Autodesk Fusion 360 part; units mm, degrees
(part 2 of 2)
sketch "Sketch2" plane through (0, 0, 11) normal (0, 0, 1) x (1, 0, 0)
  circle A0 centre (16.996833, -24.059516) radius 1
  circle A1 centre (24.059516, -16.996833) radius 1
  circle A2 centre (-20.351398, 9.391243) radius 1.05
  circle A3 centre (-9.391243, 20.351398) radius 1.05
  line L0 (24.059516, -16.996833) -> (16.996833, -24.059516) construction
  line L1 (16.996833, -24.059516) -> (15.229066, -25.827283) construction
  line L2 (24.059516, -16.996833) -> (25.827283, -15.229066) construction
  line L3 (-23.003048, 10.982233) -> (15.180718, -27.201533) construction
  line L4 (15.180718, -27.201533) -> (27.201533, -15.180718) construction
  line L5 (27.201533, -15.180718) -> (-10.982233, 23.003048) construction
  line L6 (-10.982233, 23.003048) -> (-23.003048, 10.982233)
  line L7 (-23.003048, 10.982233) -> (-31.192943, 10.982233)
  line L8 (-20.351398, 9.391243) -> (-9.391243, 20.351398) construction
  line L9 (-14.87132, 14.87132) -> (-20.284506, 20.284506) construction
  line L10 (16.996833, -24.059516) -> (18.7646, -25.827283) construction
  line L11 (25.821366, -18.770517) -> (25.827169, -18.764714) construction
  line L12 (0, 0) -> (-3.911165, 3.911165) construction
  line L13 (2.345079, -2.345079) -> (5.055897, 0.365739) construction
  arc A4 (-22.472718, 11.512563) -> (-18.056842, 7.458625) centre (-20.351398, 9.391243) ccw
  arc A5 (-7.458625, 18.056842) -> (-11.512563, 22.472718) centre (-9.391243, 20.351398) ccw
  arc A6 (25.827169, -18.764714) -> (25.827283, -15.229066) centre (24.059516, -16.996833) ccw
  arc A7 (15.229066, -25.827283) -> (18.7646, -25.827283) centre (16.996833, -24.059516) ccw
  line L14 (0, 0) -> (2.345079, -2.345079) construction
  line L15 (-8.497943, -12.497943) -> (0.242871, -12.497943)
  line L16 (12.496831, -0.24176) -> (12.496831, 8.496831)
  line L17 (8.496831, 12.496831) -> (-0.24176, 12.496831)
  line L18 (-12.497943, 0.242871) -> (-12.497943, -8.497943)
  line L19 (-12.502057, 12.502057) -> (12.502057, -12.502057) construction
  arc A8 (-12.497943, -8.497943) -> (-8.497943, -12.497943) centre (-8.497943, -8.497943) ccw
  arc A9 (12.496831, 8.496831) -> (8.496831, 12.496831) centre (8.496831, 8.496831) ccw
  line L20 (25.827283, -15.229066) -> (13.668404, -3.070187)
  line L21 (-3.070187, 13.668404) -> (-7.458625, 18.056842)
  line L22 (15.229066, -25.827283) -> (3.071298, -13.669515)
  line L23 (-13.669515, 3.071298) -> (-18.056842, 7.458625)
  arc A10 (-12.497943, 0.242871) -> (-13.669515, 3.071298) centre (-16.497943, 0.242871) ccw
  arc A11 (-3.070187, 13.668404) -> (-0.24176, 12.496831) centre (-0.24176, 16.496831) ccw
  arc A12 (12.496831, -0.24176) -> (13.668404, -3.070187) centre (16.496831, -0.24176) ccw
  arc A13 (3.071298, -13.669515) -> (0.242871, -12.497943) centre (0.242871, -16.497943) ccw
  line L24 (1.131371, -2.545584) -> (5.898877, -7.31309)
  line L25 (4.767506, -10.044461) -> (-4.767506, -10.044461)
  line L26 (0, 0) -> (-15.544001, -15.544001) construction
  arc A14 (4.767506, -10.044461) -> (5.898877, -7.31309) centre (4.767506, -8.444461) ccw
  line L27 (-5.898877, -7.31309) -> (-1.131371, -2.545584)
  arc A15 (1.131371, -2.545584) -> (-1.131371, -2.545584) centre (0, -3.676955) ccw
  arc A16 (-5.898877, -7.31309) -> (-4.767506, -10.044461) centre (-4.767506, -8.444461) ccw
  arc A17 (-2.545584, -1.131371) -> (-2.545584, 1.131371) centre (-3.676955, 0) ccw
  line L28 (-2.545584, 1.131371) -> (-7.31309, 5.898877)
  arc A18 (-7.31309, 5.898877) -> (-10.044461, 4.767506) centre (-8.444461, 4.767506) ccw
  line L29 (-10.044461, 4.767506) -> (-10.044461, -4.767506)
  arc A19 (-10.044461, -4.767506) -> (-7.31309, -5.898877) centre (-8.444461, -4.767506) ccw
  line L30 (-7.31309, -5.898877) -> (-2.545584, -1.131371)
  line L31 (7.40891, -11.085866) -> (6.847417, -11.647359)
  line L32 (6.847417, -13.910101) -> (13.99625, -21.058934)
  line L33 (16.258992, -21.058934) -> (16.820485, -20.497441)
  line L34 (16.820485, -18.234699) -> (9.671652, -11.085866)
  arc A20 (9.671652, -11.085866) -> (7.40891, -11.085866) centre (8.540281, -12.217237) ccw
  arc A21 (6.847417, -11.647359) -> (6.847417, -13.910101) centre (7.978788, -12.77873) ccw
  arc A22 (16.820485, -20.497441) -> (16.820485, -18.234699) centre (15.689114, -19.36607) ccw
  arc A23 (13.99625, -21.058934) -> (16.258992, -21.058934) centre (15.127621, -19.927563) ccw
  line L35 (-11.367395, 6.567453) -> (-10.805902, 7.128946)
  arc A24 (-10.805902, 7.128946) -> (-10.805902, 9.391688) centre (-11.937273, 8.260317) ccw
  line L36 (-10.805902, 9.391688) -> (-13.580829, 12.166615)
  arc A25 (-13.580829, 12.166615) -> (-15.843571, 12.166615) centre (-14.7122, 11.035244) ccw
  line L37 (-15.843571, 12.166615) -> (-16.405064, 11.605122)
  arc A26 (-16.405064, 11.605122) -> (-16.405064, 9.34238) centre (-15.273693, 10.473751) ccw
  line L38 (-16.405064, 9.34238) -> (-13.630137, 6.567453)
  arc A27 (-13.630137, 6.567453) -> (-11.367395, 6.567453) centre (-12.498766, 7.698824) ccw
  line L39 (18.7646, -25.827283) -> (18.770403, -25.82148)
  line L40 (25.827169, -18.764714) -> (24.412955, -20.178928) construction
  arc A28 (23.196967, -19.351249) -> (19.35125, -23.196967) centre (22.169063, -22.169063) ccw
  arc A29 (23.196967, -19.351249) -> (25.821366, -18.770517) centre (24.053713, -17.002636) ccw
  arc A30 (18.770403, -25.82148) -> (19.35125, -23.196967) centre (17.002636, -24.053713) ccw
  line L41 (0, 0) -> (31.498321, -31.498321) construction
  line L42 (-9.391688, 10.805902) -> (-12.166615, 13.580829)
  arc A31 (-12.166615, 15.843571) -> (-12.166615, 13.580829) centre (-11.035244, 14.7122) ccw
  line L43 (-12.166615, 15.843571) -> (-11.605122, 16.405064)
  arc A32 (-9.34238, 16.405064) -> (-11.605122, 16.405064) centre (-10.473751, 15.273693) ccw
  line L44 (-9.34238, 16.405064) -> (-6.567453, 13.630137)
  arc A33 (-6.567453, 11.367395) -> (-6.567453, 13.630137) centre (-7.698824, 12.498766) ccw
  line L45 (-6.567453, 11.367395) -> (-7.128946, 10.805902)
  arc A34 (-9.391688, 10.805902) -> (-7.128946, 10.805902) centre (-8.260317, 11.937273) ccw
  line L46 (-4.767506, 10.044461) -> (4.767506, 10.044461)
  arc A35 (5.898877, 7.31309) -> (4.767506, 10.044461) centre (4.767506, 8.444461) ccw
  line L47 (5.898877, 7.31309) -> (1.131371, 2.545584)
  arc A36 (-1.131371, 2.545584) -> (1.131371, 2.545584) centre (0, 3.676955) ccw
  arc A37 (-4.767506, 10.044461) -> (-5.898877, 7.31309) centre (-4.767506, 8.444461) ccw
  line L48 (-1.131371, 2.545584) -> (-5.898877, 7.31309)
  arc A38 (7.31309, -5.898877) -> (10.044461, -4.767506) centre (8.444461, -4.767506) ccw
  line L49 (10.044461, -4.767506) -> (10.044461, 4.767506)
  arc A39 (10.044461, 4.767506) -> (7.31309, 5.898877) centre (8.444461, 4.767506) ccw
  line L50 (7.31309, 5.898877) -> (2.545584, 1.131371)
  arc A40 (2.545584, 1.131371) -> (2.545584, -1.131371) centre (3.676955, 0) ccw
  line L51 (2.545584, -1.131371) -> (7.31309, -5.898877)
  line L52 (11.085866, -7.40891) -> (11.647359, -6.847417)
  arc A41 (13.910101, -6.847417) -> (11.647359, -6.847417) centre (12.77873, -7.978788) ccw
  line L53 (13.910101, -6.847417) -> (21.058934, -13.99625)
  arc A42 (21.058934, -16.258992) -> (21.058934, -13.99625) centre (19.927563, -15.127621) ccw
  line L54 (21.058934, -16.258992) -> (20.497441, -16.820485)
  arc A43 (18.234699, -16.820485) -> (20.497441, -16.820485) centre (19.36607, -15.689114) ccw
  arc A44 (11.085866, -7.40891) -> (11.085866, -9.671652) centre (12.217237, -8.540281) ccw
  line L55 (18.234699, -16.820485) -> (11.085866, -9.671652)
  line L56 (25.821366, -18.770517) -> (25.827169, -18.764714)
  point P0 (-14.87132, 14.87132)
  point P1 (-16.992641, 16.992641)
  point P2 (15.426554, -22.144069)
  point P3 (17.901428, -19.669195)
  point P4 (-0.129795, -6.58772)
  point P5 (-12.497943, -12.497943)
  point P6 (20.178814, -24.41307)
  point P7 (20.048136, -20.048136)
  dimension "d57" = 5
  dimension "d58" = 5
  dimension "d59" = 6
  dimension "d60" = 6
  dimension "d63" = 17
  dimension "d64" = 45
  dimension "d65" = 3
  dimension "d66" = 3.5
  dimension "d67" = 22
  dimension "d87" = 25
  dimension "d88" = 25
  dimension "d90" = 4
  dimension "d91" = 4
  dimension "d92" = 4
  dimension "d93" = 4
  dimension "d94" = 4
  dimension "d95" = 4
  dimension "d98" = 1.6
  dimension "d100" = 1
  dimension "d101" = 1.6
  dimension "d102" = 1.6
  dimension "d103" = 1.6
  dimension "d104" = 1.6
  dimension "d105" = 1.6
  dimension "d106" = 1.6
  dimension "d107" = 1.6
  dimension "d108" = 1.6
  dimension "d109" = 1.6
  dimension "d110" = 1.6
  dimension "d111" = 1
  dimension "d112" = 2.5
  dimension "d113" = 2.5
  dimension "d114" = 1
  dimension "d115" = 2
  dimension "d116" = 2
  dimension "d117" = 2.5
  dimension "d118" = 2.5
  constraint concentric A0 A7
  constraint concentric A1 A6
  constraint concentric A2 A4
  constraint concentric A3 A5
  constraint parallel L0 L1
  constraint parallel L0 L2
  constraint perpendicular L3 L4
  constraint parallel L3 L5
  constraint parallel L4 L6
  constraint horizontal L7
  constraint perpendicular L6 L9
  constraint tangent A7 L22
  constraint tangent A6 L20
  constraint perpendicular L1 L10
  constraint tangent L11 A6
  constraint coincident L12.start L14.start
  constraint parallel L12 L20
  constraint perpendicular L12 L13
  constraint perpendicular L13 L14
  constraint perpendicular L15 L16
  constraint parallel L15 L17
  constraint parallel L16 L18
  constraint midpoint L19 L12.start
  constraint horizontal L17
  constraint tangent L18 A8
  constraint tangent L15 A8
  constraint tangent L16 A9
  constraint tangent L17 A9
  constraint collinear L20 L21
  constraint collinear L22 L23
  constraint tangent L23 A10
  constraint tangent L18 A10
  constraint tangent L17 A11
  constraint tangent L21 A11
  constraint tangent L20 A12
  constraint tangent L16 A12
  constraint tangent L22 A13
  constraint tangent L15 A13
  constraint parallel L3 L24
  constraint perpendicular L14 L26
  constraint tangent L25 A14
  constraint tangent L24 A14
  constraint perpendicular L24 L27
  constraint tangent L24 A15
  constraint tangent L27 A15
  constraint tangent L25 A16
  constraint tangent L27 A16
  constraint symmetric L26 A14 A18
  constraint symmetric L26 A15 A17
  constraint symmetric L26 A16 A19
  constraint perpendicular L31 L32
  constraint parallel L31 L33
  constraint parallel L32 L34
  constraint perpendicular L19 L31
  constraint tangent L31 A20
  constraint tangent L34 A20
  constraint tangent L32 A21
  constraint tangent L31 A21
  constraint tangent L33 A22
  constraint tangent L34 A22
  constraint tangent L32 A23
  constraint tangent L33 A23
  constraint perpendicular L37 L38
  constraint parallel L35 L37
  constraint parallel L36 L38
  constraint tangent A25 L37
  constraint tangent L36 A25
  constraint tangent A26 L38
  constraint tangent L37 A26
  constraint tangent L35 A24
  constraint tangent A24 L36
  constraint tangent L38 A27
  constraint tangent L35 A27
  constraint tangent A7 L39
  constraint perpendicular L10 L40
  constraint tangent A28 A29
  constraint tangent L11 A29
  constraint tangent A28 A30
  constraint tangent L39 A30
  constraint perpendicular L26 L41
  constraint symmetric L19 A14 A38
  constraint symmetric L19 A15 A40
  constraint symmetric L19 A16 A39
  constraint symmetric L19 A17 A36
  constraint symmetric L19 A18 A37
  constraint symmetric L19 A19 A35
  constraint symmetric L19 A20 A44
  constraint symmetric L19 A21 A41
  constraint symmetric L19 A22 A43
  constraint symmetric L19 A23 A42
  constraint symmetric L19 A24 A34
  constraint symmetric L19 A25 A31
  constraint symmetric L19 A26 A32
  constraint symmetric L19 A27 A33
  measures "d57" diameter of A7
  measures "d58" diameter of A6
  measures "d59" diameter of A4
  measures "d60" diameter of A5
  measures "d64" angle of L3 L7
  measures "d65" distance of L6 L8
  measures "d90" radius of A8
  measures "d91" radius of A9
  measures "d92" radius of A10
  measures "d93" radius of A11
  measures "d94" radius of A12
  measures "d95" radius of A13
  measures "d98" radius of A14
  measures "d100" distance of L26 L27
  measures "d101" radius of A15
  measures "d102" radius of A16
  measures "d103" radius of A20
  measures "d104" radius of A21
  measures "d105" radius of A22
  measures "d106" radius of A23
  measures "d107" radius of A25
  measures "d108" radius of A26
  measures "d109" radius of A24
  measures "d110" radius of A27
  measures "d111" distance of L19 L34
  measures "d112" distance of L22 L32
  measures "d113" distance of L23 L38
  measures "d114" distance of L19 L36
  measures "d117" radius of A29
  measures "d118" radius of A30
extrude "Extrusion2" add sketch "Sketch2" along normal blind 2 separate body makes body 2
chamfer "Chamfer2" distance 1 angle 45 4 edges at (-21.330342, 9.770939, 13) (-10.370187, 20.731094, 13) (16.064506, -23.697901, 13) (23.127189, -16.635218, 13) on bodies 2
